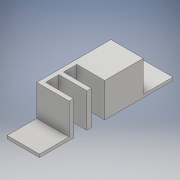
# Autodesk Inventor part: Idler Left
Saved by Autodesk Inventor 2017.3 (Build 213256000, 256)
## iProperties
Created: 2018-10-14
Part Number: Idler Left
Material: Generic
Document SubType Name: Modeling
Designer: Ax
Density: 1 g/cm^3
Appearance: Default
Author: Ax
Autodesk Inventor part; units mm, degrees
ref_plane "YZ Plane" through (0, 0, 0) normal (1, 0, 0) x (0, 1, 0)
ref_plane "XZ Plane" through (0, 0, 0) normal (0, 1, 0) x (-1, 0, 0)
ref_plane "XY Plane" through (0, 0, 0) normal (0, 0, 1) x (1, 0, 0)
sketch "Sketch3" plane through (0, 0, 0) normal (0, 0, 1) x (1, 0, 0)
  line L0 (21.8379, 25) -> (0, 25)
  line L1 (0, 25) -> (0, -25)
  line L2 (0, -25) -> (21.8379, -25)
  line L3 (21.8379, -25) -> (21.8379, -22)
  line L4 (21.8379, -22) -> (3, -22)
  line L5 (3, -22) -> (3, 22)
  line L6 (3, 22) -> (21.8379, 22)
  line L7 (21.8379, 22) -> (21.8379, 25)
  point P0 (0, 0)
  point P1 (0, 0)
  dimension "d7" = 50
  dimension "d8" = 3
  dimension "d9" = 3
  constraints: 16 end point, 7 perpendicular, 2 collinear, 1 coincident, 1 midpoint
  measures "d7" distance of L0.end L1.end
  measures "d8" distance between parallel lines of L1 L5
  measures "d9" distance of L2.end L3.end
extrude "Extrusion3" add sketch "Sketch3" along normal mid plane 23
sketch "Sketch11" plane through (0, 0, -11.5) normal (0, 0, -1) x (-1, 0, 0)
  line L0 (0, 25) -> (-21.8379, 25)
  line L1 (-21.8379, 25) -> (-21.8379, 45)
  line L2 (-21.8379, 45) -> (0, 45)
  line L3 (0, 45) -> (0, 25)
  point P0 (0, 0)
  dimension "d46" = 20
  constraints: 8 end point, 2 coincident, 2 parallel, 1 horizontal, 1 perpendicular
  measures "d46" distance of L2.end L0.start
extrude "Extrusion11" add sketch "Sketch11" against normal blind 2
mirror "Mirror1" about plane through (0, 0, 0) normal (0, 1, 0) of "Extrusion11"
sketch "Sketch13" plane through (3, -22, 11.5) normal (1, 0, 0) x (0, 0, -1)
  line L0 (0, 47) -> (0, -3) projected
  line L1 (23, -23) -> (23, 67) projected
  line L2 (0, 12) -> (23, 12)
  line L3 (23, 12) -> (23, 9)
  line L4 (23, 9) -> (0, 9)
  line L5 (0, 9) -> (0, 12)
  line L6 (23, 0) -> (0, 0) projected
  line L7 (23, 44) -> (0, 44) projected
  line L8 (0, 44) -> (23, 44)
  line L9 (23, 44) -> (23, 21)
  line L10 (23, 21) -> (0, 21)
  line L11 (0, 21) -> (0, 44)
  point P0 (11.5, 22)
  dimension "d57" = 9
  dimension "d58" = 3
  dimension "d62" = 9
  constraints: 16 end point, 4 parallel, 3 point on line, 2 horizontal, 2 perpendicular
  measures "d57" distance between parallel lines of L4 L6
  measures "d58" distance between parallel lines of L2 L4
  measures "d62" distance between parallel lines of L2 L10
extrude "Extrusion12" add sketch "Sketch13" along normal up to surface (18.8379 mm away) contours L7 L1 L10 L0 | L2 L1 L4 L0
body "Solid2"
